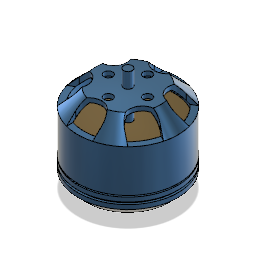
motor v5 (Autodesk Fusion 360 design; units mm, degrees)
Autodesk Fusion 360 part; units mm, degrees
note: some values were not read from the file. Set by a fixed rule: which sketch regions a step uses.
sketch "Sketch1" plane through (0, 0, 0) normal (0, 0, 1) x (1, 0, 0)
  line L0 (0, 18.1387) -> (0, -5.6613)
  line L1 (0, -5.6613) -> (1, -5.6613)
  line L2 (1, -5.6613) -> (1, -3.8613)
  line L3 (1, -3.8613) -> (9.5, -3.8613)
  line L4 (9.5, -3.8613) -> (11.5, -1.8613)
  line L5 (11.5, 10.6387) -> (7.5, 14.6387)
  line L6 (7.5, 14.6387) -> (1, 14.6387)
  line L7 (1, 14.6387) -> (1, 18.1387)
  line L8 (1, 18.1387) -> (0, 18.1387)
  line L9 (2, 13.6387) -> (7.0858, 13.6387)
  line L10 (7.0858, 13.6387) -> (10.5, 10.2245)
  line L11 (10.5, 10.2245) -> (10.5, 7.9809)
  line L12 (10.5, 7.9809) -> (1, 7.9809)
  line L13 (1, 7.9809) -> (1, 12.6387)
  line L14 (1, 12.6387) -> (2, 12.6387)
  line L15 (2, 12.6387) -> (2, 13.6387)
  line L16 (11.5, -0.8613) -> (11, -0.8613)
  line L17 (11, -0.8613) -> (11, -0.3613)
  line L18 (11, -0.3613) -> (11.5, -0.3613)
  line L19 (11.5, 0.6387) -> (9.5, 0.6387)
  line L20 (9.5, 0.6387) -> (9.5, 0.9387)
  line L21 (9.5, 0.9387) -> (11.5, 0.9387)
  line L22 (11.5, -1.8613) -> (11.5, -0.8613)
  line L23 (11.5, -0.3613) -> (11.5, 0.6387)
  line L24 (11.5, 0.9387) -> (11.5, 10.6387)
  dimension "d5" = 23.8
  dimension "d6" = 1.8
  dimension "d7" = 45
  dimension "d8" = 2
  dimension "d9" = 11.5
  dimension "d10" = 1
  dimension "d11" = 1
  dimension "d12" = 3.5
  dimension "d14" = 4
  dimension "d15" = 1
  dimension "d17" = 1
  dimension "d18" = 1
  dimension "d19" = 1
  dimension "d20" = 1
  dimension "d21" = 1
  dimension "d22" = 0.5
  dimension "d23" = 0.5
  dimension "d24" = 1
  dimension "d25" = 2
  dimension "d26" = 0.3
  dimension "d27" = 1
  constraint vertical L0
  constraint perpendicular L0 L1
  constraint perpendicular L1 L2
  constraint perpendicular L2 L3
  constraint parallel L2 L22
  constraint perpendicular L4 L5
  constraint perpendicular L6 L22
  constraint perpendicular L6 L7
  constraint perpendicular L0 L8
  constraint coincident origin L0
  constraint perpendicular L7 L9
  constraint perpendicular L9 L11
  constraint perpendicular L11 L12
  constraint perpendicular L9 L13
  constraint perpendicular L13 L14
  constraint perpendicular L9 L15
  constraint parallel L5 L10
  constraint perpendicular L16 L22
  constraint perpendicular L16 L17
  constraint coincident L18.end L22
  constraint perpendicular L18 L22
  constraint coincident L19.start L22
  constraint perpendicular L19 L22
  constraint perpendicular L19 L20
  constraint coincident L21.end L22
  constraint perpendicular L21 L22
  constraint collinear L22 L23
  constraint collinear L23 L24
  measures "d5" distance of L0.start L0.end
  measures "d6" distance of L1.end L2.end
  measures "d7" angle of L3 L4
  measures "d8" vertical distance of L3.end L4.end
  measures "d9" distance of L0 L22
  measures "d10" distance of L0.start L7.end
  measures "d11" distance of L0.end L1.end
  measures "d12" distance of L6.end L7.end
  measures "d14" vertical distance of L5.start L5.end
  measures "d15" distance of L6 L9
  measures "d17" distance of L11 L22
  measures "d18" distance of L0 L13
  measures "d19" distance of L5 L10
  measures "d20" distance of L14.end L9.start
  measures "d21" distance of L13.end L14.end
  measures "d22" distance of L17.end L18.end
  measures "d23" distance of L16.end L17.end
  measures "d24" distance of L4.end L16.start
  measures "d25" distance of L20.end L21.end
  measures "d26" distance of L19.end L20.end
  measures "d27" distance of L18.end L19.start
revolve "Revolve1" add sketch "Sketch1" angle 360 about axis through (0, 18.1387, 0) along (0, -1, 0)
sketch "Sketch2" plane through (0, 14.6387, 0) normal (0, 1, 0) x (-1, 0, 0)
  circle A0 centre (0, 0) radius 1
  circle A1 centre (0, 0) radius 7.5
  circle A2 centre (0, 0) radius 4.5 construction
  circle A3 centre (0, 0) radius 8.5777 construction
  line L0 (0, 0) -> (0, -9) construction
  circle A4 centre (0, 4.5) radius 1
  circle A5 centre (-4.5, 0) radius 1
  circle A6 centre (0, -4.5) radius 1
  circle A7 centre (4.5, 0) radius 1
  line L1 (3, -9) -> (3, -15.6157)
  line L2 (-3, -9) -> (-3, -15.6157)
  line L3 (-3, -15.6157) -> (3, -15.6157)
  arc A8 (3, -9) -> (-3, -9) centre (0, -9) ccw
  line L4 (9.2942, -1.9019) -> (15.0236, -5.2098)
  arc A9 (9.2942, -1.9019) -> (6.2942, -7.0981) centre (7.7942, -4.5) ccw
  line L5 (6.2942, -7.0981) -> (12.0236, -10.4059)
  line L6 (12.0236, -10.4059) -> (15.0236, -5.2098)
  line L7 (6.2942, 7.0981) -> (12.0236, 10.4059)
  arc A10 (6.2942, 7.0981) -> (9.2942, 1.9019) centre (7.7942, 4.5) ccw
  line L8 (9.2942, 1.9019) -> (15.0236, 5.2098)
  line L9 (15.0236, 5.2098) -> (12.0236, 10.4059)
  line L10 (-3, 9) -> (-3, 15.6157)
  arc A11 (-3, 9) -> (3, 9) centre (0, 9) ccw
  line L11 (3, 9) -> (3, 15.6157)
  line L12 (3, 15.6157) -> (-3, 15.6157)
  line L13 (-9.2942, 1.9019) -> (-15.0236, 5.2098)
  arc A12 (-9.2942, 1.9019) -> (-6.2942, 7.0981) centre (-7.7942, 4.5) ccw
  line L14 (-6.2942, 7.0981) -> (-12.0236, 10.4059)
  line L15 (-12.0236, 10.4059) -> (-15.0236, 5.2098)
  line L16 (-6.2942, -7.0981) -> (-12.0236, -10.4059)
  arc A13 (-6.2942, -7.0981) -> (-9.2942, -1.9019) centre (-7.7942, -4.5) ccw
  line L17 (-9.2942, -1.9019) -> (-15.0236, -5.2098)
  line L18 (-15.0236, -5.2098) -> (-12.0236, -10.4059)
  dimension "d29" = 9
  dimension "d30" = 9
  dimension "d31" = 2
  dimension "d33" = 360
  dimension "d34" = 6
  dimension "d36" = 360
  constraint concentric A0 A2
  constraint coincident A0.centre A1.centre
  constraint vertical L0
  constraint coincident A2 A4.centre
  constraint coincident L0.end A8.centre
  constraint parallel L0 L1
  constraint parallel L1 L2
  constraint perpendicular L1 L3
  constraint tangent L1 A8
  constraint tangent L2 A8
  measures "d29" diameter of A2
  measures "d30" distance of A0.centre L0.end
  measures "d31" diameter of A4
  measures "d34" diameter of A8
extrude "Extrude1" cut sketch "Sketch2" against normal blind 4 contours A1 A10 | A1 L7 A10 L8 L9 | A1 L4 A9 L5 L6 | A1 A9 | A1 A11 | A1 L10 A11 L11 L12 | A1 L1 L2 L3 A8 | A1 A8 | A1 A12 | A1 L13 A12 L14 L15 | A1 L16 A13 L17 L18 | A1 A13 | A4 | A5 | A6 | A7
sketch "Sketch3" plane through (0, -3.8613, 0) normal (0, -1, 0) x (1, 0, 0)
  circle A0 centre (0, 0) radius 9.5
  circle A1 centre (0, 0) radius 1
  circle A2 centre (0, 0) radius 8 construction
  circle A3 centre (0, 0) radius 6 construction
  circle A4 centre (0, 6) radius 1
  circle A5 centre (0, -6) radius 1
  circle A6 centre (8, 0) radius 1
  dimension "d39" = 12
  dimension "d40" = 16
  constraint coincident A0.centre A1.centre
  constraint concentric A0 A3
  constraint coincident A3 A4.centre
  constraint coincident A3 A5.centre
  constraint coincident A2 A6.centre
  constraint equal A4 A6
  constraint equal A5 A6
  measures "d39" diameter of A3
  measures "d40" diameter of A2
extrude "Extrude2" cut sketch "Sketch3" against normal blind 3 contours A4 | A5 | A6
